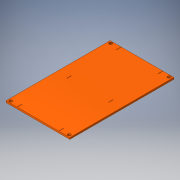
# Autodesk Inventor part: LCD_PCB
Saved by Autodesk Inventor 2016 (Build 200138000, 138)
## iProperties
Created: 2016-04-06
Part Number: LCD_PCB
Material: Phenolic Resin
Document SubType Name: Modeling
Designer: agmle
Mass: 12.983 g
Surface Area: 122.656 cm^2
Volume: 9.408 cm^3
Density: 1.38 g/cm^3
Appearance: Smooth - Light Orange
Author: agmle
Autodesk Inventor part; units mm, degrees
ref_plane "YZ Plane" through (0, 0, 0) normal (1, 0, 0) x (0, 1, 0)
ref_plane "XZ Plane" through (0, 0, 0) normal (0, 1, 0) x (-1, 0, 0)
ref_plane "XY Plane" through (0, 0, 0) normal (0, 0, 1) x (1, 0, 0)
sketch "Sketch1" plane through (0, 0, 0) normal (0, 1, 0) x (-1, 0, 0)
  line L0 (36.5132, 47.4786) -> (-23.4868, 47.4786)
  line L1 (-23.4868, 47.4786) -> (-23.4868, -50.5214)
  line L2 (-23.4868, -50.5214) -> (36.5132, -50.5214)
  line L3 (36.5132, -50.5214) -> (36.5132, 47.4786)
  point P0 (0, 0)
  dimension "d0" = 98
  dimension "d1" = 60
  constraints: 8 end point, 2 parallel, 1 horizontal, 1 perpendicular
  measures "d0" distance of L2.end L0.start
  measures "d1" distance of L0.start L0.end
extrude "Extrusion1" add sketch "Sketch1" along normal blind 1.6
sketch "Sketch2" plane through (0, 1.6, 0) normal (0, 1, 0) x (1, 0, 0)
  line L0 (-26.2632, -46.9786) -> (13.2368, -46.9786) construction
  line L1 (13.2368, -46.9786) -> (13.2368, 50.0214) construction
  line L2 (13.2368, 50.0214) -> (-26.2632, 50.0214) construction
  line L3 (-26.2632, 50.0214) -> (-26.2632, -46.9786) construction
  line L4 (-36.5132, 50.5214) -> (-36.5132, -47.4786) construction
  line L5 (-36.5132, 1.5214) -> (-26.2632, 1.5214) construction
  line L6 (13.2368, 1.5214) -> (23.4868, 1.5214) construction
  line L7 (23.4868, -47.4786) -> (23.4868, 50.5214) construction
  line L8 (-26.2632, -46.9786) -> (-26.0132, -46.9786)
  line L9 (-26.0132, -46.9786) -> (-26.0132, -42.9786)
  line L10 (-26.0132, -42.9786) -> (-26.2632, -42.9786)
  line L11 (-26.2632, -42.9786) -> (-26.2632, -46.9786)
  line L12 (-26.2632, -0.4786) -> (-26.0132, -0.4786)
  line L13 (-26.0132, -0.4786) -> (-26.0132, 3.5214)
  line L14 (-26.0132, 3.5214) -> (-26.2632, 3.5214)
  line L15 (-26.2632, 3.5214) -> (-26.2632, -0.4786)
  line L16 (-26.2632, 46.0214) -> (-26.0132, 46.0214)
  line L17 (-26.0132, 46.0214) -> (-26.0132, 50.0214)
  line L18 (-26.0132, 50.0214) -> (-26.2632, 50.0214)
  line L19 (-26.2632, 50.0214) -> (-26.2632, 46.0214)
  line L20 (12.9868, 46.0214) -> (13.2368, 46.0214)
  line L21 (13.2368, 46.0214) -> (13.2368, 50.0214)
  line L22 (13.2368, 50.0214) -> (12.9868, 50.0214)
  line L23 (12.9868, 50.0214) -> (12.9868, 46.0214)
  line L24 (12.9868, 3.5214) -> (13.2368, 3.5214)
  line L25 (13.2368, 3.5214) -> (13.2368, -0.4786)
  line L26 (13.2368, -0.4786) -> (12.9868, -0.4786)
  line L27 (12.9868, -0.4786) -> (12.9868, 3.5214)
  line L28 (12.9868, -46.9786) -> (13.2368, -46.9786)
  line L29 (13.2368, -46.9786) -> (13.2368, -42.9786)
  line L30 (13.2368, -42.9786) -> (12.9868, -42.9786)
  line L31 (12.9868, -42.9786) -> (12.9868, -46.9786)
  line L32 (-26.1382, -42.9786) -> (-26.1382, -0.4786) construction
  line L33 (-26.1382, 3.5214) -> (-26.1382, 46.0214) construction
  point P0 (0, 0)
  dimension "d4" = 39.5
  dimension "d5" = 97
  dimension "d6" = 0.25
  dimension "d7" = 4
  constraints: 64 end point, 14 parallel, 13 point on line, 8 midpoint, 7 horizontal, 7 perpendicular, 6 equal length, 5 collinear
  measures "d4" distance of L0.start L0.end
  measures "d5" distance of L2.end L0.start
  measures "d6" distance of L9.end L10.end
  measures "d7" distance of L8.end L9.end
extrude "Extrusion2" cut sketch "Sketch2" against normal blind 1.6
sketch "Sketch3" plane through (0, 1.6, 0) normal (0, 1, 0) x (1, 0, 0)
  line L0 (-36.5132, -47.4786) -> (23.4868, -47.4786) projected
  line L1 (-34.0132, -45.4786) -> (20.9868, -45.4786) construction
  line L2 (20.9868, -45.4786) -> (20.9868, 48.5214) construction
  line L3 (20.9868, 48.5214) -> (-34.0132, 48.5214) construction
  line L4 (-34.0132, 48.5214) -> (-34.0132, -45.4786) construction
  line L5 (23.4868, 50.5214) -> (-36.5132, 50.5214) construction
  line L6 (-36.5132, 50.5214) -> (-36.5132, -47.4786) construction
  point P0 (0, 0)
  dimension "d10" = 2
  dimension "d11" = 55
  dimension "d12" = 2
  dimension "d13" = 2.5
  constraints: 8 end point, 2 perpendicular, 1 parallel, 1 vertical
  measures "d10" distance from line of L0 L1.start
  measures "d11" distance of L1.end L1.start
  measures "d12" distance from line of L5 L3.end
  measures "d13" distance between parallel lines of L6 L4
hole "Hole1" at (-34.0132, 1.6, 45.4786) at (-34.0132, 1.6, -48.5214) at (20.9868, 1.6, -48.5214) at (20.9868, 1.6, 45.4786) direction (0, -1, 0) diameter 3 end through all
body "Solid1"
